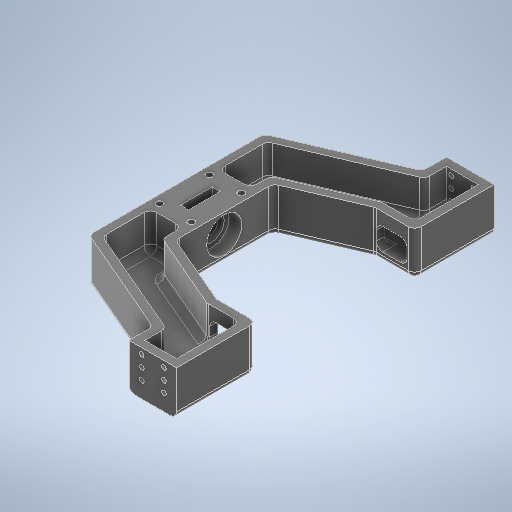
# Autodesk Inventor part: wahacz_tylny
Saved by Autodesk Inventor 2025.2 (Build 292293000, 293)
## iProperties
Created: 2026-04-18
Part Number: wahacz_tylny
Material: PCTG 20%
Document SubType Name: Modeling
Designer: ksawe
Density: 1.541 g/cm^3
Appearance: Smooth - Black
Author: ksawe
Autodesk Inventor part; units mm, degrees
ref_plane "YZ Plane" through (0, 0, 0) normal (1, 0, 0) x (0, 1, 0)
sketch "Sketch1" plane through (0, 0, 0) normal (0, 1, 0) x (-1, 0, 0)
  line L0 (-100, 100) -> (-70, 100)
  line L1 (0, 0) -> (-70, 0) construction
  line L2 (-100, 100) -> (-100, 50)
  line L3 (-100, 50) -> (-75, 50)
  line L4 (-70, 100) -> (-70, 85)
  line L5 (-70, 85) -> (0, 55)
  line L6 (0, 55) -> (0, 0)
  line L7 (-75, 50) -> (-30, 30.7143)
  line L8 (-30, 30.7143) -> (-30, 0)
  line L9 (-100, -100) -> (-70, -100)
  line L10 (-100, -100) -> (-100, -50)
  line L11 (-100, -50) -> (-75, -50)
  line L12 (-70, -100) -> (-70, -85)
  line L13 (-70, -85) -> (0, -55)
  line L14 (0, -55) -> (0, 0)
  line L15 (-75, -50) -> (-30, -30.7143)
  line L16 (-30, -30.7143) -> (-30, 0)
  line L17 (-5, 0) -> (-5, 51.703)
  line L18 (-5, 51.703) -> (-75, 81.703)
  line L19 (-75, 81.703) -> (-75, 95)
  line L20 (-75, 95) -> (-95, 95)
  line L21 (-95, 95) -> (-95, 55)
  line L22 (-95, 55) -> (-73.9737, 55)
  line L23 (-73.9737, 55) -> (-25, 34.0113)
  line L24 (-25, 34.0113) -> (-25, 0)
  line L25 (-25, 0) -> (-25, -34.0113)
  line L26 (-25, -34.0113) -> (-73.9737, -55)
  line L27 (-73.9737, -55) -> (-95, -55)
  line L28 (-95, -55) -> (-95, -95)
  line L29 (-95, -95) -> (-75, -95)
  line L30 (-75, -95) -> (-75, -81.703)
  line L31 (-75, -81.703) -> (-5, -51.703)
  line L32 (-5, -51.703) -> (-5, 0)
  dimension "d0" = 100
  dimension "d5" = 30
  dimension "d20" = 50
  dimension "d21" = 25
  dimension "d23" = 15
  dimension "d26" = 100
  dimension "d27" = 55
  dimension "d29" = 30
  dimension "d32" = 70
  dimension "d33" = 5
  constraints: 66 end point, 7 symmetric about line, 4 coincident, 4 vertical, 2 horizontal, 2 parallel, 1 horizontal alignment, 15 other
  measures "d0" distance between parallel lines of L1 L0
  measures "d5" distance of L0.start L0.end
  measures "d20" distance of L0.start L2.end
  measures "d21" distance of L2.end L3.end
  measures "d23" distance of L0.end L4.end
  measures "d26" distance between parallel lines of L2 L6
  measures "d27" distance of L5.end L6.end
  measures "d29" distance between parallel lines of L8 L6
  measures "d32" distance of L1.start L1.end
  measures "d33" distance between parallel lines of L6 L17
extrude "Extrusion3" add sketch "Sketch1" against normal blind 6 contours L0 L4 L5 L6 L14 L13 L12 L9 L10 L11 L15 L16 L8 L7 L3 L2 | L32 L31 L30 L29 L28 L27 L26 L25 L24 L23 L22 L21 L20 L19 L18 L17
extrude "Extrusion4" add sketch "Sketch1" along normal blind 22
sketch "Szkic3" plane through (0, 0, 0) normal (0, 1, 0) x (1, 0, 0)
  line L0 (25.5, 10) -> (4.5, 10)
  line L1 (4.5, 10) -> (4.5, -10)
  line L2 (4.5, -10) -> (25.5, -10)
  line L3 (25.5, -10) -> (25.5, 10)
  line L4 (25.5, 10) -> (4.5, -10) construction
  line L5 (4.5, 10) -> (25.5, -10) construction
  line L6 (5, -51.703) -> (5, 51.703) projected
  line L7 (5, -21.5) -> (25, -21.5)
  line L8 (25, -34.0113) -> (25, 34.0113) projected
  line L9 (5, 21.5) -> (25, 21.5)
  line L10 (5, 0) -> (25, 0) construction
  line L11 (17.5, -10) -> (17.5, 10)
  line L12 (12.5, 10) -> (12.5, -10)
  point P0 (0, 0)
  point P1 (15, 0)
  point P2 (5, 10)
  point P3 (25, 10)
  point P4 (25, -10)
  point P5 (5, -10)
  dimension "d34" = 21
  dimension "d35" = 10
  dimension "d36" = 20
  dimension "d37" = 11.5
  dimension "d96" = 7.5
  dimension "d97" = 7.5
  constraints: 22 end point, 8 point on line, 4 midpoint, 4 perpendicular, 2 horizontal, 2 parallel, 1 horizontal alignment, 1 other
  measures "d34" distance of L2.end L1.end
  measures "d35" distance from line of L6 point (15, 0)
  measures "d36" distance between parallel lines of L0 L2
  measures "d37" distance between parallel lines of L2 L7
  measures "d96" distance between parallel lines of L12 L6
  measures "d97" distance between parallel lines of L8 L11
extrude "Wyciągnięcie proste6" add sketch "Szkic3" along normal blind 22 contours L0 L6 L9 L8 | L0 L8 L2 L11 | L12 L2 L6 L0 | L2 L8 L7 L6
sketch "Szkic4" plane through (30, -6, 30.7143) normal (1, 0, 0) x (0, 0, -1)
  circle A0 centre (30.7143, 15.5) radius 6
  circle A1 centre (30.7143, 15.5) radius 11.05
  line L0 (61.4286, 0) -> (61.4286, 28) projected
  line L1 (61.4286, 0) -> (0, 0) projected
  point P0 (30.7143, 6)
  dimension "d40" = 12
  dimension "d41" = 22.1
  dimension "d103" = 15.5
  constraints: 2 centre point, 2 coincident, 1 vertical alignment
  measures "d40" diameter of A0
  measures "d41" diameter of A1
  measures "d103" distance from line of L1 A0.centre
extrude "Wyciągnięcie proste7" cut sketch "Szkic4" against normal blind 8
extrude "Wyciągnięcie proste8" cut sketch "Szkic4" against normal through all contours A0
sketch "Szkic9" plane through (0, 22, 0) normal (0, 1, 0) x (1, 0, 0)
  circle A0 centre (5, -15.75) radius 1.5
  line L0 (5, -21.5) -> (25, -21.5) projected
  line L1 (0, 55) -> (0, -55) projected
  line L2 (25, 21.5) -> (5, 21.5) projected
  line L3 (15, -21.5) -> (15, 21.5)
  line L4 (0, 0) -> (30, 0)
  line L5 (30, 30.7143) -> (30, -30.7143) projected
  circle A1 centre (25, -15.75) radius 1.5
  circle A2 centre (5, 15.75) radius 1.5
  circle A3 centre (25, 15.75) radius 1.5
  dimension "d52" = 3
  dimension "d98" = 5.75
  dimension "d99" = 5
  constraints: 4 centre point, 4 end point, 4 midpoint, 3 symmetric about line, 3 other
  measures "d52" diameter of A0
  measures "d98" distance from line of L0 A0.centre
  measures "d99" distance from line of L1 A0.centre
hole "Otwór1" at (5, 22, 15.75) at (25, 22, 15.75) at (25, 22, -15.75) at (5, 22, -15.75) direction (0, -1, 0) diameter 4 depth 7 countersink diameter 4.2 countersink angle 90
sketch "Szkic10" plane through (95, 0, 95) normal (0, 0, -1) x (-1, 0, 0)
  circle A0 centre (3, 18.25) radius 1.5
  line L0 (0, 0) -> (0, 22) projected
  line L1 (0, 22) -> (20, 22) projected
  circle A1 centre (17, 18.25) radius 1.5
  circle A2 centre (3, 11.25) radius 1.5
  circle A3 centre (17, 11.25) radius 1.5
  circle A4 centre (3, 4.25) radius 1.5
  circle A5 centre (17, 4.25) radius 1.5
  line L2 (10, 22) -> (10, 0) construction
  line L3 (20, 0) -> (0, 0) projected
  point P0 (95, 0)
  dimension "d60" = 3
  dimension "d64" = 14
  dimension "d67" = 7
  dimension "d70" = 3.75
  constraints: 6 centre point, 2 end point, 2 midpoint, 1 horizontal, 1 vertical, 11 other
  measures "d60" diameter of A0
  measures "d64" distance of A0.centre A1.centre
  measures "d67" distance of A0.centre A2.centre
  measures "d70" distance from line of L1 A0.centre
extrude "Wyciągnięcie proste11" cut sketch "Szkic10" against normal through all
fillet "Zaokrąglenie1" radius 4 50 edges at (0, -6, 0) (35, -6, -70) (30, -6, 0) (52.5, -6, -40.3571) (52.5, -6, 40.3571) (35, -6, 70) (87.5, -6, -50) (100, -6, -75) (70, -6, -92.5) (87.5, -6, 50) (100, -6, 75) (70, -6, 92.5) (0, 8, 55) (0, 8, -55) (70, 8, -85) (70, 8, 85) (30, 8, -30.7143) (30, 8, 30.7143) (75, 8, 50) (75, 8, -50) (100, 8, -50) (100, 8, 50) (5, 11, -51.703) (5, 11, 51.703) (73.9737, 11, 55) (25, 11, 34.0113) (25, 11, -34.0113) (73.9737, 11, -55) (5, 11, -21.5) (25, 11, -21.5) (25, 0, -27.7556) (49.4869, 0, -44.5056) (5, 0, -36.6015) (40, 0, -66.703) (5, 0, 36.6015) (15, 0, 21.5) (40, 0, 66.703) (25, 0, 27.7556) (49.4869, 0, 44.5056) (5, 11, 21.5) (25, 11, 21.5) (84.4869, 0, 55) (95, 0, 75) (75, 0, 88.3515) (75, 11, 81.703) (75, 11, -81.703) (75, 0, -88.3515) (95, 0, -75) (84.4869, 0, -55) (95, 11, -55)
fillet "Zaokrąglenie2" radius 4 2 edges at (93.8284, 1.1716, 56.1716) (95, 13, 55)
sketch "Sketch12" plane through (96, 22, 50) normal (0, 0, -1) x (-1, 0, 0)
  arc A0 (1, -18) -> (5, -22) centre (5, -18) ccw projected
  line L0 (21.2053, -22) -> (5, -22) projected
  line L1 (21.2053, -18) -> (21.2053, 0) projected
  line L2 (20.179, 0) -> (20.179, -24) projected
  line L3 (1, -18) -> (1, 0) projected
  line L4 (1, -8) -> (20.179, -8)
  line L5 (0, 0) -> (20.179, 0) projected
  point P0 (96, -22)
  point P1 (20.179, -22)
  dimension "d90" = 8
  constraints: 2 end point, 2 point on line, 1 perpendicular
  measures "d90" distance between parallel lines of L5 L4
extrude "Extrusion15" cut sketch "Sketch12" against normal blind 9 contours L3 L4 L2 L0 A0
fillet "Fillet3" radius 4 3 edges at (75.821, 14, 52.5) (95, 14, 54.5) (75.821, 0, 54.5)
ref_plane "Work Plane4" through (15, 0, 10) normal (1, 0, 0) x (0, 0, -1)
mirror "Mirror4" about plane through (15, 0, 10) normal (1, 0, 0) of "Wyciągnięcie proste7"
ref_plane "Work Plane5" through (9, 22, 0) normal (0, 0, 1) x (1, 0, 0)
mirror "Mirror5" about plane through (9, 22, 0) normal (0, 0, 1) of "Extrusion15", "Wyciągnięcie proste11", "Fillet3"
fillet "Fillet4" radius 2 2 edges at (22, 9.5, 6) (8, 9.5, 6)
body "Solid2"
